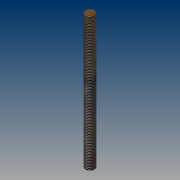
# Autodesk Inventor part: BOLT
Saved by Autodesk Inventor 2014 (Build 180170000, 170)
## iProperties
Created: 2021-03-21
Part Number: BOLT
Material: Stainless Steel
Document SubType Name: Modeling
Designer: Think Station
Density: 8.08 g/cm^3
Appearance: Small Uneven Rectanguler Stones - Brown
Mass: 95.1903 g
Surface Area: 48.6947 cm^2
Volume: 11.781 cm^3
Author: Think Station
Autodesk Inventor part; units mm, degrees
ref_plane "YZ Plane" through (0, 0, 0) normal (1, 0, 0) x (0, 1, 0)
ref_plane "XZ Plane" through (0, 0, 0) normal (0, 1, 0) x (-1, 0, 0)
ref_plane "XY Plane" through (0, 0, 0) normal (0, 0, 1) x (1, 0, 0)
sketch "Sketch1" plane through (0, 0, 0) normal (0, 0, 1) x (1, 0, 0)
  circle A0 centre (0, 0) radius 5
  dimension "d0" = 10
  constraints: 1 centre point, 1 coincident
  measures "d0" diameter of A0
extrude "Extrusion1" add sketch "Sketch1" along normal blind 150
thread "Thread1" size "M10x1.5" class "6g" standard "ANSI Metric M Profile" full length
body "Solid1"
